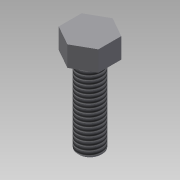
# Autodesk Inventor part: Болт М5х16
Saved by Autodesk Inventor 2018 (Build 220112000, 112)
## iProperties
Created: 2020-03-16
Part Number: Болт М5х16
Material: Типовые
Document SubType Name: Modeling
Designer: Leancher
Density: 1 g/cm^3
Appearance: По умолчанию
Author: Leancher
Autodesk Inventor part; units mm, degrees
ref_plane "YZ Plane" through (0, 0, 0) normal (1, 0, 0) x (0, 1, 0)
ref_plane "XZ Plane" through (0, 0, 0) normal (0, 1, 0) x (-1, 0, 0)
ref_plane "XY Plane" through (0, 0, 0) normal (0, 0, 1) x (1, 0, 0)
sketch "Эскиз1" plane through (0, 0, 0) normal (0, 0, 1) x (1, 0, 0)
  line L0 (0, -4.45) -> (-3.9, -2.2517)
  line L1 (3.9, -2.2517) -> (0, -4.45)
  line L2 (0, 4.45) -> (3.9, 2.2517)
  line L3 (-3.9, 2.2517) -> (0, 4.45)
  line L4 (-3.9, -2.2517) -> (-3.9, 2.2517)
  line L5 (3.9, -2.2517) -> (3.9, 2.2517)
  point P0 (0, 0)
  constraints: 12 end point, 1 point on line
extrude "Выдавливание1" add sketch "Эскиз1" along normal blind 4
sketch "Эскиз2" plane through (0, 0, 0) normal (0, 0, -1) x (-1, 0, 0)
  circle A0 centre (0, 0) radius 2.4
  dimension "d2" = 4.8
  constraints: 1 centre point, 1 coincident
  measures "d2" diameter of A0
extrude "Выдавливание2" add sketch "Эскиз2" along normal blind 16
thread "Резьба1" size "M5x0.8" class "6g" standard "ANSI Metric M Profile" full length
chamfer "Фаска1" distance 0.3 angle 45 1 edges at (2.4, 0, -16)
